Autodesk Fusion 360 part; units mm, degrees
note: some values were not read from the file. Set by a fixed rule: which sketch regions a step uses.
(part 4 of 5)
  spline S974 degree 3 poles (-10.77395, -44.821587) (-10.585081, -45.023839) (-10.376922, -45.203062) (-10.149782, -45.360193) knots 0 0 0 0 1 1 1 1
  spline S975 degree 3 poles (-10.149782, -45.359877) (-9.922331, -45.517324) (-9.680879, -45.648629) (-9.425424, -45.753798) knots 0 0 0 0 1 1 1 1
  spline S976 degree 3 poles (-9.425424, -45.753482) (-9.169969, -45.858967) (-8.906426, -45.936132) (-8.63448, -45.984667) knots 0 0 0 0 1 1 1 1
  spline S977 degree 3 poles (-8.63448, -45.984667) (-8.383382, -46.030411) (-8.130417, -46.050946) (-7.875585, -46.046586) knots 0 0 0 0 1 1 1 1
  spline S978 degree 3 poles (-7.875585, -46.046586) (-7.62013, -46.04099) (-7.368098, -46.010808) (-7.119178, -45.955112) knots 0 0 0 0 1 1 1 1
  spline S979 degree 3 poles (-7.119178, -45.955112) (-6.869947, -45.899727) (-6.628805, -45.820073) (-6.395754, -45.716149) knots 0 0 0 0 1 1 1 1
  spline S980 degree 3 poles (-6.395754, -45.716149) (-6.162391, -45.612225) (-5.942097, -45.486209) (-5.733937, -45.338101) knots 0 0 0 0 1 1 1 1
  spline S981 degree 3 poles (-5.733937, -45.338101) (-5.522666, -45.186571) (-5.328197, -45.016061) (-5.150219, -44.826259) knots 0 0 0 0 1 1 1 1
  spline S982 degree 3 poles (-5.150219, -44.826259) (-4.972552, -44.636457) (-4.814799, -44.431098) (-4.67727, -44.210181) knots 0 0 0 0 1 1 1 1
  spline S983 degree 3 poles (-4.67727, -44.210181) (-4.540053, -43.989265) (-4.425238, -43.757147) (-4.333449, -43.513827) knots 0 0 0 0 1 1 1 1
  spline S984 degree 3 poles (-4.333449, -43.513827) (-4.24166, -43.270196) (-4.174451, -43.020343) (-4.131824, -42.763644) knots 0 0 0 0 1 1 1 1
  spline S985 degree 3 poles (-4.131824, -42.763644) (-4.031011, -42.270782) (-3.876369, -41.795655) (-3.66821, -41.337953) knots 0 0 0 0 1 1 1 1
  spline S986 degree 3 poles (-3.66821, -41.337953) (-3.46005, -40.87994) (-3.203351, -40.451486) (-2.898113, -40.051658) knots 0 0 0 0 1 1 1 1
  line L17 (-2.898113, -40.051658) -> (-2.628968, -39.723701)
  spline S987 degree 3 poles (-2.628968, -39.723701) (-2.587897, -39.676095) (-2.537801, -39.641557) (-2.478683, -39.62071) knots 0 0 0 0 1 1 1 1
  spline S988 degree 3 poles (-2.478683, -39.62071) (-2.419564, -39.599863) (-2.35889, -39.595195) (-2.297282, -39.607019) knots 0 0 0 0 1 1 1 1
  spline S989 degree 3 poles (-11.970634, -36.872008) (-11.933296, -36.878851) (-11.898136, -36.890988) (-11.865154, -36.908724) knots 0 0 0 0 1 1 1 1
  spline S990 degree 3 poles (-11.865154, -36.908724) (-11.831861, -36.926771) (-11.802301, -36.949485) (-11.776476, -36.976866) knots 0 0 0 0 1 1 1 1
  spline S991 degree 3 poles (-11.776476, -36.976866) (-11.75065, -37.004247) (-11.729492, -37.035051) (-11.713623, -37.069277) knots 0 0 0 0 1 1 1 1
  spline S992 degree 3 poles (-11.713623, -37.069277) (-11.697444, -37.103504) (-11.687176, -37.139286) (-11.68282, -37.176624) knots 0 0 0 0 1 1 1 1
  line L18 (-11.68282, -37.176624) -> (-11.521333, -38.552842)
  spline S993 degree 3 poles (-11.521333, -38.552842) (-11.49893, -39.47478) (-11.568316, -40.389873) (-11.729181, -41.298121) knots 0 0 0 0 1 1 1 1
  line L19 (-11.729181, -41.298121) -> (-11.758429, -41.485433)
  spline S994 degree 3 poles (-11.758429, -41.485433) (-11.837772, -41.923533) (-11.842128, -42.362255) (-11.770564, -42.80191) knots 0 0 0 0 1 1 1 1
  spline S995 degree 3 poles (-11.770564, -42.80191) (-11.76745, -42.824313) (-11.766518, -42.847027) (-11.768386, -42.869119) knots 0 0 0 0 1 1 1 1
  spline S996 degree 3 poles (-11.768386, -42.869119) (-11.769002, -42.892455) (-11.772427, -42.914858) (-11.778028, -42.93695) knots 0 0 0 0 1 1 1 1
  spline S997 degree 3 poles (-11.778654, -42.936327) (-11.783627, -42.959041) (-11.791096, -42.980511) (-11.801053, -43.001047) knots 0 0 0 0 1 1 1 1
  spline S998 degree 3 poles (-11.801368, -43.000113) (-11.810699, -43.021582) (-11.822211, -43.041185) (-11.835591, -43.059543) knots 0 0 0 0 1 1 1 1
  spline S999 degree 3 poles (-11.835591, -43.059543) (-11.849281, -43.077901) (-11.864216, -43.094703) (-11.881645, -43.109327) knots 0 0 0 0 1 1 1 1
  spline S1000 degree 3 poles (-11.881645, -43.109327) (-11.897821, -43.125507) (-11.915867, -43.139197) (-11.93547, -43.151021) knots 0 0 0 0 1 1 1 1
  spline S1001 degree 3 poles (-11.93547, -43.151021) (-11.954761, -43.162845) (-11.975297, -43.172801) (-11.997081, -43.179958) knots 0 0 0 0 1 1 1 1
  spline S1002 degree 3 poles (-11.997081, -43.179958) (-12.017925, -43.18867) (-12.039705, -43.194582) (-12.062108, -43.198005) knots 0 0 0 0 1 1 1 1
  spline S1003 degree 3 poles (-12.062734, -43.197382) (-12.084511, -43.201741) (-12.107225, -43.203294) (-12.129939, -43.202672) knots 0 0 0 0 1 1 1 1
  spline S1004 degree 3 poles (-12.129939, -43.202672) (-12.152653, -43.201741) (-12.175056, -43.198936) (-12.197147, -43.19396) knots 0 0 0 0 1 1 1 1
  spline S1005 degree 3 poles (-12.197147, -43.19396) (-12.21955, -43.18867) (-12.241019, -43.181514) (-12.261555, -43.17249) knots 0 0 0 0 1 1 1 1
  spline S1006 degree 3 poles (-12.261555, -43.17249) (-12.282402, -43.163156) (-12.302005, -43.151954) (-12.320674, -43.138886) knots 0 0 0 0 1 1 1 1
  spline S1007 degree 3 poles (-12.320674, -43.138886) (-12.339343, -43.125818) (-12.356456, -43.111194) (-12.372325, -43.094703) knots 0 0 0 0 1 1 1 1
  spline S1008 degree 3 poles (-12.372325, -43.094703) (-12.387882, -43.078212) (-12.402195, -43.060476) (-12.414956, -43.040563) knots 0 0 0 0 1 1 1 1
  spline S1009 degree 3 poles (-12.414956, -43.040563) (-12.426776, -43.022205) (-12.437044, -43.00198) (-12.445445, -42.980822) knots 0 0 0 0 1 1 1 1
  spline S1010 degree 3 poles (-12.445445, -42.980822) (-12.453846, -42.959664) (-12.460069, -42.937883) (-12.464114, -42.91548) knots 0 0 0 0 1 1 1 1
  spline S1011 degree 3 poles (-12.464114, -42.91548) (-12.548747, -42.399593) (-12.545013, -41.884639) (-12.452605, -41.369997) knots 0 0 0 0 1 1 1 1
  line L20 (-12.452605, -41.369997) -> (-12.424602, -41.188285)
  spline S1012 degree 3 poles (-12.424602, -41.188285) (-12.271827, -40.3348) (-12.204307, -39.47478) (-12.221732, -38.607916) knots 0 0 0 0 1 1 1 1
  line L21 (-12.221732, -38.607916) -> (-12.383219, -37.259701)
  spline S1013 degree 3 poles (-12.383219, -37.259701) (-12.386333, -37.23232) (-12.386644, -37.204939) (-12.383537, -37.177869) knots 0 0 0 0 1 1 1 1
  spline S1014 degree 3 poles (-12.383537, -37.177869) (-12.380423, -37.150488) (-12.374203, -37.123729) (-12.364557, -37.097903) knots 0 0 0 0 1 1 1 1
  spline S1015 degree 3 poles (-12.364557, -37.097903) (-12.355223, -37.072078) (-12.343088, -37.047497) (-12.327841, -37.024472) knots 0 0 0 0 1 1 1 1
  spline S1016 degree 3 poles (-12.327841, -37.024472) (-12.312906, -37.001447) (-12.295482, -36.9806) (-12.275257, -36.961619) knots 0 0 0 0 1 1 1 1
  spline S1017 degree 3 poles (-12.275257, -36.961619) (-12.255343, -36.942639) (-12.233252, -36.926459) (-12.209604, -36.912769) knots 0 0 0 0 1 1 1 1
  spline S1018 degree 3 poles (-12.209604, -36.912769) (-12.185646, -36.898767) (-12.160754, -36.888188) (-12.134306, -36.880409) knots 0 0 0 0 1 1 1 1
  spline S1019 degree 3 poles (-12.134306, -36.880409) (-12.107858, -36.872319) (-12.081099, -36.867652) (-12.053718, -36.866096) knots 0 0 0 0 1 1 1 1
  spline S1020 degree 3 poles (-12.053718, -36.866096) (-12.026026, -36.864543) (-11.998956, -36.866415) (-11.971885, -36.871075) knots 0 0 0 0 1 1 1 1
  line L22 (-11.971885, -36.871075) -> (-11.970634, -36.872008)
  spline S1021 degree 3 poles (-10.675626, -35.450051) (-10.638599, -35.456583) (-10.603439, -35.46872) (-10.570457, -35.486456) knots 0 0 0 0 1 1 1 1
  spline S1022 degree 3 poles (-10.570457, -35.486456) (-10.537475, -35.504191) (-10.507916, -35.526905) (-10.482091, -35.553976) knots 0 0 0 0 1 1 1 1
  spline S1023 degree 3 poles (-10.482091, -35.553976) (-10.456265, -35.581357) (-10.435418, -35.611849) (-10.419238, -35.646076) knots 0 0 0 0 1 1 1 1
  spline S1024 degree 3 poles (-10.419238, -35.646076) (-10.403058, -35.679991) (-10.39279, -35.715463) (-10.388123, -35.752801) knots 0 0 0 0 1 1 1 1
  line L23 (-10.388123, -35.752801) -> (-10.25215, -36.838404)
  spline S1025 degree 3 poles (-10.25215, -36.838404) (-10.073861, -38.475054) (-10.114622, -40.106104) (-10.375052, -41.732173) knots 0 0 0 0 1 1 1 1
  spline S1026 degree 3 poles (-10.375052, -41.732173) (-10.388434, -41.811208) (-10.39808, -41.891173) (-10.403682, -41.971761) knots 0 0 0 0 1 1 1 1
  spline S1027 degree 3 poles (-10.403989, -41.972381) (-10.409281, -42.052349) (-10.411146, -42.132937) (-10.408971, -42.213525) knots 0 0 0 0 1 1 1 1
  spline S1028 degree 3 poles (-10.408968, -42.214145) (-10.406797, -42.294113) (-10.40057, -42.374701) (-10.390614, -42.454667) knots 0 0 0 0 1 1 1 1
  spline S1029 degree 3 poles (-10.39061, -42.455286) (-10.380346, -42.534943) (-10.366344, -42.614287) (-10.348608, -42.693008) knots 0 0 0 0 1 1 1 1
  spline S1030 degree 3 poles (-10.348605, -42.693628) (-10.330562, -42.771729) (-10.309092, -42.849205) (-10.283578, -42.925748) knots 0 0 0 0 1 1 1 1
  spline S1031 degree 3 poles (-10.283574, -42.926368) (-10.258064, -43.002291) (-10.228815, -43.077589) (-10.195834, -43.151332) knots 0 0 0 0 1 1 1 1
  spline S1032 degree 3 poles (-10.19583, -43.151952) (-10.162852, -43.224764) (-10.126447, -43.296639) (-10.08662, -43.366959) knots 0 0 0 0 1 1 1 1
  spline S1033 degree 3 poles (-10.086616, -43.367579) (-10.046793, -43.436968) (-10.003543, -43.504799) (-9.95687, -43.570763) knots 0 0 0 0 1 1 1 1
  spline S1034 degree 3 poles (-9.956866, -43.571383) (-9.910198, -43.636727) (-9.860413, -43.69989) (-9.807518, -43.760876) knots 0 0 0 0 1 1 1 1
  spline S1035 degree 3 poles (-9.807825, -43.761495) (-9.754622, -43.821861) (-9.698926, -43.880046) (-9.64043, -43.935431) knots 0 0 0 0 1 1 1 1
  spline S1036 degree 3 poles (-9.640738, -43.936362) (-9.581934, -43.991127) (-9.520949, -44.0434) (-9.457163, -44.092873) knots 0 0 0 0 1 1 1 1
  spline S1037 degree 3 poles (-9.457159, -44.093493) (-9.393377, -44.142346) (-9.327413, -44.188396) (-9.259271, -44.231335) knots 0 0 0 0 1 1 1 1
  spline S1038 degree 3 poles (-9.259267, -44.232266) (-9.190818, -44.274273) (-9.120809, -44.31379) (-9.048622, -44.349883) knots 0 0 0 0 1 1 1 1
  spline S1039 degree 3 poles (-9.048619, -44.350503) (-8.976436, -44.385976) (-8.902693, -44.418336) (-8.827395, -44.446962) knots 0 0 0 0 1 1 1 1
  spline S1040 degree 3 poles (-8.827702, -44.447893) (-8.752096, -44.475899) (-8.675553, -44.500791) (-8.597766, -44.52226) knots 0 0 0 0 1 1 1 1
  spline S1041 degree 3 poles (-8.598073, -44.52288) (-8.519978, -44.543418) (-8.441568, -44.560843) (-8.361914, -44.574222) knots 0 0 0 0 1 1 1 1
  spline S1042 degree 3 poles (-8.362221, -44.574842) (-8.28257, -44.587602) (-8.202605, -44.597247) (-8.122017, -44.602848) knots 0 0 0 0 1 1 1 1
  spline S1043 degree 3 poles (-8.122324, -44.603779) (-8.04174, -44.608449) (-7.961152, -44.610311) (-7.880564, -44.608138) knots 0 0 0 0 1 1 1 1
  spline S1044 degree 3 poles (-7.880872, -44.608758) (-7.799978, -44.605653) (-7.7197, -44.599426) (-7.639734, -44.589158) knots 0 0 0 0 1 1 1 1
  spline S1045 degree 3 poles (-7.640041, -44.590089) (-7.559768, -44.579201) (-7.480425, -44.564888) (-7.402014, -44.547152) knots 0 0 0 0 1 1 1 1
  spline S1046 degree 3 poles (-7.402011, -44.547772) (-7.323293, -44.529106) (-7.245818, -44.507325) (-7.169275, -44.4815) knots 0 0 0 0 1 1 1 1
  spline S1047 degree 3 poles (-7.169582, -44.482431) (-7.093043, -44.455985) (-7.017744, -44.426737) (-6.944313, -44.393755) knots 0 0 0 0 1 1 1 1
  spline S1048 degree 3 poles (-6.94431, -44.394375) (-6.87057, -44.360773) (-6.799006, -44.324058) (-6.728996, -44.28423) knots 0 0 0 0 1 1 1 1
  spline S1049 degree 3 poles (-6.728993, -44.28485) (-6.658988, -44.244092) (-6.591157, -44.200531) (-6.525194, -44.153858) knots 0 0 0 0 1 1 1 1
  spline S1050 degree 3 poles (-6.525502, -44.154478) (-6.459541, -44.107186) (-6.396066, -44.057402) (-6.335392, -44.004195) knots 0 0 0 0 1 1 1 1
  spline S1051 degree 3 poles (-6.335389, -44.005126) (-6.274406, -43.951299) (-6.216221, -43.895604) (-6.160837, -43.836796) knots 0 0 0 0 1 1 1 1
  spline S1052 degree 3 poles (-6.161145, -43.837416) (-6.105452, -43.777989) (-6.053179, -43.717003) (-6.003706, -43.652906) knots 0 0 0 0 1 1 1 1
  spline S1053 degree 3 poles (-6.004014, -43.653837) (-5.954545, -43.589121) (-5.908494, -43.523157) (-5.865555, -43.454704) knots 0 0 0 0 1 1 1 1
  spline S1054 degree 3 poles (-5.865552, -43.455323) (-5.822616, -43.386251) (-5.7831, -43.315931) (-5.747007, -43.243744) knots 0 0 0 0 1 1 1 1
  spline S1055 degree 3 poles (-5.747315, -43.244364) (-5.711224, -43.171557) (-5.678865, -43.097814) (-5.649928, -43.022205) knots 0 0 0 0 1 1 1 1
  spline S1056 degree 3 poles (-5.650237, -43.022825) (-5.621301, -42.946906) (-5.596409, -42.870052) (-5.575252, -42.792265) knots 0 0 0 0 1 1 1 1
  spline S1057 degree 3 poles (-5.575249, -42.792885) (-5.553782, -42.714477) (-5.536668, -42.635756) (-5.522978, -42.556102) knots 0 0 0 0 1 1 1 1
  spline S1058 degree 3 poles (-5.523287, -42.556721) (-5.431811, -42.127959) (-5.309218, -41.709151) (-5.15551, -41.299366) knots 0 0 0 0 1 1 1 1
  spline S1059 degree 3 poles (-5.155819, -41.299985) (-5.001802, -40.889892) (-4.818845, -40.493797) (-4.606019, -40.111083) knots 0 0 0 0 1 1 1 1
  spline S1060 degree 3 poles (-4.606327, -40.111391) (-4.393503, -39.728679) (-4.153917, -39.364011) (-3.887261, -39.017389) knots 0 0 0 0 1 1 1 1
  spline S1061 degree 3 poles (-3.887259, -39.017698) (-3.620294, -38.670768) (-3.329369, -38.345616) (-3.014171, -38.042242) knots 0 0 0 0 1 1 1 1
  spline S1062 degree 3 poles (-3.014171, -38.042242) (-2.997994, -38.025753) (-2.980258, -38.011129) (-2.961276, -37.99837) knots 0 0 0 0 1 1 1 1
  spline S1063 degree 3 poles (-2.961276, -37.99837) (-2.941987, -37.985304) (-2.921762, -37.974414) (-2.90029, -37.965699) knots 0 0 0 0 1 1 1 1
  spline S1064 degree 3 poles (-2.90029, -37.965699) (-2.879134, -37.956678) (-2.857043, -37.949833) (-2.834638, -37.945474) knots 0 0 0 0 1 1 1 1
  spline S1065 degree 3 poles (-2.834638, -37.945474) (-2.811926, -37.940809) (-2.788901, -37.938634) (-2.765873, -37.93832) knots 0 0 0 0 1 1 1 1
  spline S1066 degree 3 poles (-2.765873, -37.93832) (-2.742851, -37.938323) (-2.719826, -37.940498) (-2.69742, -37.945163) knots 0 0 0 0 1 1 1 1
  spline S1067 degree 3 poles (-2.69742, -37.945163) (-2.674709, -37.949522) (-2.652617, -37.956056) (-2.631145, -37.964766) knots 0 0 0 0 1 1 1 1
  spline S1068 degree 3 poles (-2.631145, -37.964766) (-2.609989, -37.973791) (-2.589765, -37.98437) (-2.570471, -37.997125) knots 0 0 0 0 1 1 1 1
  spline S1069 degree 3 poles (-2.570471, -37.997125) (-2.551182, -38.010196) (-2.533447, -38.024509) (-2.516953, -38.040997) knots 0 0 0 0 1 1 1 1
  spline S1070 degree 3 poles (-2.516953, -38.040997) (-2.500776, -38.05718) (-2.486152, -38.074915) (-2.473081, -38.094204) knots 0 0 0 0 1 1 1 1
  spline S1071 degree 3 poles (-2.473081, -38.094204) (-2.460326, -38.113187) (-2.449436, -38.133723) (-2.440721, -38.154878) knots 0 0 0 0 1 1 1 1
  spline S1072 degree 3 poles (-2.440721, -38.154878) (-2.4317, -38.17635) (-2.424855, -38.198131) (-2.420497, -38.220842) knots 0 0 0 0 1 1 1 1
  spline S1073 degree 3 poles (-2.420497, -38.220842) (-2.415832, -38.243559) (-2.413654, -38.266584) (-2.413651, -38.289606) knots 0 0 0 0 1 1 1 1
  spline S1074 degree 3 poles (-2.413651, -38.289606) (-2.413343, -38.312634) (-2.415521, -38.335659) (-2.420185, -38.358371) knots 0 0 0 0 1 1 1 1
  spline S1075 degree 3 poles (-2.420185, -38.358371) (-2.424544, -38.381087) (-2.431078, -38.402868) (-2.440099, -38.424334) knots 0 0 0 0 1 1 1 1
  spline S1076 degree 3 poles (-2.440099, -38.424334) (-2.448814, -38.445806) (-2.459393, -38.466031) (-2.472459, -38.48532) knots 0 0 0 0 1 1 1 1
  spline S1077 degree 3 poles (-2.472459, -38.48532) (-2.485218, -38.504614) (-2.499531, -38.522349) (-2.51602, -38.538838) knots 0 0 0 0 1 1 1 1
  spline S1078 degree 3 poles (-2.51602, -38.538838) (-2.804458, -38.817009) (-3.070803, -39.114779) (-3.315676, -39.43215) knots 0 0 0 0 1 1 1 1
  spline S1079 degree 3 poles (-3.315676, -39.43215) (-3.560554, -39.749526) (-3.780848, -40.083079) (-3.976559, -40.43281) knots 0 0 0 0 1 1 1 1
  spline S1080 degree 3 poles (-3.976559, -40.43281) (-4.172586, -40.782545) (-4.341852, -41.144724) (-4.484668, -41.519346) knots 0 0 0 0 1 1 1 1
  spline S1081 degree 3 poles (-4.484668, -41.519346) (-4.627488, -41.893974) (-4.742302, -42.277) (-4.829111, -42.668424) knots 0 0 0 0 1 1 1 1
  spline S1082 degree 3 poles (-4.829111, -42.668424) (-4.846227, -42.770795) (-4.868629, -42.871919) (-4.895697, -42.972107) knots 0 0 0 0 1 1 1 1
  spline S1083 degree 3 poles (-4.895697, -42.972107) (-4.92277, -43.0723) (-4.954818, -43.170935) (-4.991843, -43.2677) knots 0 0 0 0 1 1 1 1
  spline S1084 degree 3 poles (-4.991843, -43.2677) (-5.028561, -43.364781) (-5.069944, -43.459682) (-5.116303, -43.552714) knots 0 0 0 0 1 1 1 1
  spline S1085 degree 3 poles (-5.116303, -43.552714) (-5.162355, -43.64575) (-5.213073, -43.735983) (-5.268144, -43.824037) knots 0 0 0 0 1 1 1 1
  spline S1086 degree 3 poles (-5.268144, -43.824037) (-5.322909, -43.911783) (-5.382339, -43.997039) (-5.4455, -44.07918) knots 0 0 0 0 1 1 1 1
  spline S1087 degree 3 poles (-5.4455, -44.07918) (-5.508978, -44.161326) (-5.576186, -44.240047) (-5.647436, -44.315654) knots 0 0 0 0 1 1 1 1
  spline S1088 degree 3 poles (-5.647436, -44.315654) (-5.718381, -44.390955) (-5.793058, -44.462831) (-5.871153, -44.53097) knots 0 0 0 0 1 1 1 1
  spline S1089 degree 3 poles (-5.871153, -44.53097) (-5.949256, -44.599114) (-6.030777, -44.663522) (-6.115095, -44.723572) knots 0 0 0 0 1 1 1 1
  spline S1090 degree 3 poles (-6.115095, -44.723572) (-6.199421, -44.783627) (-6.286854, -44.839634) (-6.376772, -44.891282) knots 0 0 0 0 1 1 1 1
  spline S1091 degree 3 poles (-6.376772, -44.891282) (-6.466699, -44.942935) (-6.558799, -44.989919) (-6.653386, -45.032544) knots 0 0 0 0 1 1 1 1
  spline S1092 degree 3 poles (-6.653386, -45.032544) (-6.747978, -45.074863) (-6.844124, -45.112824) (-6.942444, -45.145803) knots 0 0 0 0 1 1 1 1
  spline S1093 degree 3 poles (-6.942444, -45.145803) (-7.040771, -45.178787) (-7.140339, -45.207102) (-7.24146, -45.230125) knots 0 0 0 0 1 1 1 1
  spline S1094 degree 3 poles (-7.24146, -45.230125) (-7.342275, -45.253463) (-7.444333, -45.271821) (-7.547009, -45.284887) knots 0 0 0 0 1 1 1 1
  spline S1095 degree 3 poles (-7.547009, -45.284887) (-7.649692, -45.298269) (-7.752994, -45.306359) (-7.856603, -45.309468) knots 0 0 0 0 1 1 1 1
  spline S1096 degree 3 poles (-7.856603, -45.309468) (-7.96022, -45.312584) (-8.063522, -45.310402) (-8.16682, -45.303247) knots 0 0 0 0 1 1 1 1
  spline S1097 degree 3 poles (-8.16682, -45.303247) (-8.270438, -45.296089) (-8.373116, -45.283959) (-8.47517, -45.266843) knots 0 0 0 0 1 1 1 1
  spline S1098 degree 3 poles (-8.47517, -45.266843) (-8.577542, -45.249732) (-8.678666, -45.227329) (-8.778542, -45.200257) knots 0 0 0 0 1 1 1 1
  spline S1099 degree 3 poles (-8.778542, -45.200257) (-8.878424, -45.173189) (-8.977059, -45.141141) (-9.073823, -45.104422) knots 0 0 0 0 1 1 1 1
  spline S1100 degree 3 poles (-9.073823, -45.104422) (-9.170595, -45.067398) (-9.265495, -45.026015) (-9.358215, -44.979651) knots 0 0 0 0 1 1 1 1
  spline S1101 degree 3 poles (-9.358215, -44.979651) (-9.450941, -44.933603) (-9.541175, -44.882886) (-9.628915, -44.82781) knots 0 0 0 0 1 1 1 1
  spline S1102 degree 3 poles (-9.628915, -44.82781) (-9.716974, -44.772739) (-9.801607, -44.71362) (-9.883747, -44.650143) knots 0 0 0 0 1 1 1 1
  spline S1103 degree 3 poles (-9.883747, -44.650143) (-9.965584, -44.586671) (-10.044305, -44.519462) (-10.11991, -44.448206) knots 0 0 0 0 1 1 1 1
  spline S1104 degree 3 poles (-10.11991, -44.448206) (-10.195212, -44.377267) (-10.266777, -44.302591) (-10.334914, -44.224178) knots 0 0 0 0 1 1 1 1
  spline S1105 degree 3 poles (-10.334914, -44.224178) (-10.40306, -44.146082) (-10.466845, -44.064561) (-10.526894, -43.980236) knots 0 0 0 0 1 1 1 1
  spline S1106 degree 3 poles (-10.526894, -43.980236) (-10.586949, -43.895606) (-10.642956, -43.808484) (-10.694293, -43.718248) knots 0 0 0 0 1 1 1 1
  spline S1107 degree 3 poles (-10.694293, -43.718248) (-10.745947, -43.628328) (-10.792931, -43.535916) (-10.835244, -43.441324) knots 0 0 0 0 1 1 1 1
  spline S1108 degree 3 poles (-10.835244, -43.441324) (-10.877564, -43.346737) (-10.915213, -43.25028) (-10.948191, -43.151954) knots 0 0 0 0 1 1 1 1
  spline S1109 degree 3 poles (-10.948191, -43.151954) (-10.981177, -43.053633) (-11.009492, -42.953754) (-11.032513, -42.852628) knots 0 0 0 0 1 1 1 1
  spline S1110 degree 3 poles (-11.032513, -42.852628) (-11.055542, -42.751506) (-11.0739, -42.649449) (-11.086964, -42.546456) knots 0 0 0 0 1 1 1 1
  spline S1111 degree 3 poles (-11.086964, -42.546456) (-11.100036, -42.443779) (-11.108126, -42.340477) (-11.111234, -42.23655) knots 0 0 0 0 1 1 1 1
  spline S1112 degree 3 poles (-11.111234, -42.23655) (-11.114352, -42.13294) (-11.11217, -42.029327) (-11.105013, -41.925711) knots 0 0 0 0 1 1 1 1
  spline S1113 degree 3 poles (-11.105013, -41.925711) (-11.097864, -41.822412) (-11.085726, -41.719421) (-11.068609, -41.61705) knots 0 0 0 0 1 1 1 1
  spline S1114 degree 3 poles (-11.068609, -41.61705) (-10.819692, -40.059434) (-10.780798, -38.496837) (-10.95162, -36.928951) knots 0 0 0 0 1 1 1 1
  line L24 (-10.95162, -36.928951) -> (-11.0879, -35.84054)
  spline S1115 degree 3 poles (-11.0879, -35.84054) (-11.090704, -35.81752) (-11.091325, -35.794495) (-11.089765, -35.771465) knots 0 0 0 0 1 1 1 1
  spline S1116 degree 3 poles (-11.089765, -35.771465) (-11.088211, -35.748444) (-11.084165, -35.72573) (-11.078252, -35.703323) knots 0 0 0 0 1 1 1 1
  spline S1117 degree 3 poles (-11.078252, -35.703323) (-11.072032, -35.681236) (-11.063939, -35.659767) (-11.05336, -35.638915) knots 0 0 0 0 1 1 1 1
  spline S1118 degree 3 poles (-11.05336, -35.638915) (-11.043092, -35.618384) (-11.030957, -35.598781) (-11.016644, -35.580418) knots 0 0 0 0 1 1 1 1
  spline S1119 degree 3 poles (-11.016644, -35.580418) (-11.002643, -35.562377) (-10.986774, -35.545574) (-10.969349, -35.530323) knots 0 0 0 0 1 1 1 1
  spline S1120 degree 3 poles (-10.969349, -35.530323) (-10.951925, -35.515393) (-10.932945, -35.502013) (-10.913031, -35.490496) knots 0 0 0 0 1 1 1 1
  spline S1121 degree 3 poles (-10.913031, -35.490496) (-10.893118, -35.479299) (-10.871959, -35.469654) (-10.850179, -35.462492) knots 0 0 0 0 1 1 1 1
  spline S1122 degree 3 poles (-10.850179, -35.462492) (-10.828087, -35.455035) (-10.805684, -35.450051) (-10.78297, -35.447246) knots 0 0 0 0 1 1 1 1
  spline S1123 degree 3 poles (-10.78297, -35.447246) (-10.746877, -35.442584) (-10.711095, -35.443515) (-10.675626, -35.450051) knots 0 0 0 0 1 1 1 1
  spline S1124 degree 3 poles (-5.153642, -34.44877) (-5.0883, -34.460593) (-5.030738, -34.488597) (-4.980953, -34.533091) knots 0 0 0 0 1 1 1 1
  spline S1125 degree 3 poles (-4.980953, -34.533091) (-4.931481, -34.577586) (-4.897254, -34.631726) (-4.878585, -34.695512) knots 0 0 0 0 1 1 1 1
  spline S1126 degree 3 poles (-4.878585, -34.695512) (-4.859605, -34.759609) (-4.858983, -34.823706) (-4.876407, -34.887803) knots 0 0 0 0 1 1 1 1
  spline S1127 degree 3 poles (-4.876407, -34.887803) (-4.894143, -34.952211) (-4.927124, -35.007284) (-4.975975, -35.052712) knots 0 0 0 0 1 1 1 1
  spline S1128 degree 3 poles (-4.975975, -35.052712) (-5.485639, -35.502947) (-5.956098, -35.991142) (-6.387042, -36.517297) knots 0 0 0 0 1 1 1 1
  spline S1129 degree 3 poles (-6.387042, -36.517297) (-6.817984, -37.043452) (-7.204122, -37.601033) (-7.546388, -38.189421) knots 0 0 0 0 1 1 1 1
  spline S1130 degree 3 poles (-7.546388, -38.189421) (-7.886474, -38.778115) (-8.178334, -39.390459) (-8.420719, -40.026139) knots 0 0 0 0 1 1 1 1
  spline S1131 degree 3 poles (-8.421342, -40.026141) (-8.663416, -40.661819) (-8.853218, -41.313056) (-8.990747, -41.979231) knots 0 0 0 0 1 1 1 1
  spline S1132 degree 3 poles (-8.990747, -41.979231) (-9.003192, -42.047682) (-9.009104, -42.116446) (-9.00786, -42.185835) knots 0 0 0 0 1 1 1 1
  spline S1133 degree 3 poles (-9.00786, -42.185835) (-9.006927, -42.254908) (-8.999147, -42.323672) (-8.984524, -42.391506) knots 0 0 0 0 1 1 1 1
  spline S1134 degree 3 poles (-8.984524, -42.391506) (-8.969899, -42.459334) (-8.949052, -42.524987) (-8.921672, -42.588464) knots 0 0 0 0 1 1 1 1
  spline S1135 degree 3 poles (-8.921672, -42.588464) (-8.893978, -42.652247) (-8.860685, -42.71261) (-8.82117, -42.769553) knots 0 0 0 0 1 1 1 1
  spline S1136 degree 3 poles (-8.82117, -42.769553) (-8.781964, -42.826802) (-8.73747, -42.879387) (-8.687687, -42.927617) knots 0 0 0 0 1 1 1 1
  spline S1137 degree 3 poles (-8.687687, -42.927617) (-8.637902, -42.975843) (-8.584073, -43.018782) (-8.525889, -43.056434) knots 0 0 0 0 1 1 1 1
  spline S1138 degree 3 poles (-8.525889, -43.056434) (-8.467702, -43.09408) (-8.406406, -43.125507) (-8.341999, -43.151023) knots 0 0 0 0 1 1 1 1
  spline S1139 degree 3 poles (-8.341999, -43.151023) (-8.27759, -43.176535) (-8.211315, -43.195515) (-8.143174, -43.207964) knots 0 0 0 0 1 1 1 1
  spline S1140 degree 3 poles (-8.143174, -43.207964) (-8.075031, -43.220407) (-8.006267, -43.226319) (-7.937192, -43.225077) knots 0 0 0 0 1 1 1 1
  spline S1141 degree 3 poles (-7.937192, -43.225077) (-7.867805, -43.223833) (-7.799352, -43.216051) (-7.731522, -43.20143) knots 0 0 0 0 1 1 1 1
  spline S1142 degree 3 poles (-7.731522, -43.20143) (-7.664001, -43.186803) (-7.598348, -43.165645) (-7.534564, -43.138266) knots 0 0 0 0 1 1 1 1
  spline S1143 degree 3 poles (-7.534564, -43.138266) (-7.471088, -43.110571) (-7.410725, -43.076967) (-7.353786, -43.037765) knots 0 0 0 0 1 1 1 1
  spline S1144 degree 3 poles (-7.353786, -43.037765) (-7.296844, -42.998246) (-7.244259, -42.953441) (-7.196034, -42.903659) knots 0 0 0 0 1 1 1 1
  spline S1145 degree 3 poles (-7.196034, -42.903659) (-7.147803, -42.853872) (-7.105175, -42.799732) (-7.067528, -42.74155) knots 0 0 0 0 1 1 1 1
  spline S1146 degree 3 poles (-7.067528, -42.74155) (-7.029878, -42.683362) (-6.998451, -42.621754) (-6.972938, -42.557349) knots 0 0 0 0 1 1 1 1
  spline S1147 degree 3 poles (-6.972938, -42.557349) (-6.947422, -42.492938) (-6.928442, -42.426352) (-6.915998, -42.358212) knots 0 0 0 0 1 1 1 1
  spline S1148 degree 3 poles (-6.915998, -42.358212) (-6.801181, -41.805296) (-6.642495, -41.265139) (-6.439316, -40.738053) knots 0 0 0 0 1 1 1 1
  spline S1149 degree 3 poles (-6.439316, -40.738053) (-6.237066, -40.210962) (-5.993124, -39.703787) (-5.70811, -39.216526) knots 0 0 0 0 1 1 1 1
  spline S1150 degree 3 poles (-5.707179, -39.216528) (-5.422786, -38.729264) (-5.100123, -38.268139) (-4.740122, -37.833463) knots 0 0 0 0 1 1 1 1
  spline S1151 degree 3 poles (-4.740122, -37.833463) (-4.37981, -37.398474) (-3.986827, -36.995846) (-3.561173, -36.625266) knots 0 0 0 0 1 1 1 1
  spline S1152 degree 3 poles (-3.561173, -36.625266) (-3.54406, -36.61002) (-3.525702, -36.59664) (-3.5061, -36.585128) knots 0 0 0 0 1 1 1 1
  spline S1153 degree 3 poles (-3.5061, -36.585128) (-3.486186, -36.573615) (-3.46565, -36.564281) (-3.44387, -36.556813) knots 0 0 0 0 1 1 1 1
  spline S1154 degree 3 poles (-3.44387, -36.556813) (-3.4224, -36.549032) (-3.400309, -36.543745) (-3.377595, -36.540633) knots 0 0 0 0 1 1 1 1
  spline S1155 degree 3 poles (-3.377595, -36.540633) (-3.355192, -36.537519) (-3.332478, -36.536586) (-3.309453, -36.537838) knots 0 0 0 0 1 1 1 1
  spline S1156 degree 3 poles (-3.309453, -36.537838) (-3.286739, -36.538769) (-3.264336, -36.542505) (-3.242244, -36.548106) knots 0 0 0 0 1 1 1 1
  spline S1157 degree 3 poles (-3.242244, -36.548106) (-3.220153, -36.553706) (-3.198683, -36.561174) (-3.178147, -36.571131) knots 0 0 0 0 1 1 1 1
  spline S1158 degree 3 poles (-3.178147, -36.571131) (-3.1573, -36.580776) (-3.138009, -36.5926) (-3.119651, -36.606291) knots 0 0 0 0 1 1 1 1
  spline S1159 degree 3 poles (-3.119651, -36.606291) (-3.101293, -36.61967) (-3.08418, -36.634916) (-3.068934, -36.65203) knots 0 0 0 0 1 1 1 1
  spline S1160 degree 3 poles (-3.068934, -36.65203) (-3.053687, -36.668832) (-3.039997, -36.68719) (-3.028173, -36.706481) knots 0 0 0 0 1 1 1 1
  spline S1161 degree 3 poles (-3.028173, -36.706481) (-3.016349, -36.726084) (-3.006393, -36.746619) (-2.998614, -36.768089) knots 0 0 0 0 1 1 1 1
  spline S1162 degree 3 poles (-2.998614, -36.768089) (-2.990835, -36.789558) (-2.984923, -36.81165) (-2.981501, -36.834364) knots 0 0 0 0 1 1 1 1
  spline S1163 degree 3 poles (-2.981501, -36.834364) (-2.978078, -36.856767) (-2.976522, -36.879481) (-2.977456, -36.902506) knots 0 0 0 0 1 1 1 1
  spline S1164 degree 3 poles (-2.977456, -36.902506) (-2.978389, -36.92522) (-2.981501, -36.947934) (-2.98679, -36.970025) knots 0 0 0 0 1 1 1 1
  spline S1165 degree 3 poles (-2.98679, -36.970025) (-2.99208, -36.992428) (-2.999236, -37.013898) (-3.008882, -37.034745) knots 0 0 0 0 1 1 1 1
  spline S1166 degree 3 poles (-3.008882, -37.034745) (-3.018216, -37.055592) (-3.029729, -37.075194) (-3.042797, -37.093863) knots 0 0 0 0 1 1 1 1
  spline S1167 degree 3 poles (-3.042797, -37.093863) (-3.056177, -37.112532) (-3.071112, -37.129645) (-3.087603, -37.145203) knots 0 0 0 0 1 1 1 1
  spline S1168 degree 3 poles (-3.087603, -37.145203) (-3.482452, -37.49058) (-3.847121, -37.865205) (-4.181918, -38.269389) knots 0 0 0 0 1 1 1 1
  spline S1169 degree 3 poles (-4.181918, -38.269389) (-4.516405, -38.673262) (-4.816976, -39.101094) (-5.08239, -39.55319) knots 0 0 0 0 1 1 1 1
  spline S1170 degree 3 poles (-5.08239, -39.55319) (-5.349354, -40.005296) (-5.57805, -40.475756) (-5.768785, -40.964573) knots 0 0 0 0 1 1 1 1
  spline S1171 degree 3 poles (-5.768476, -40.964568) (-5.959831, -41.45339) (-6.11074, -41.954342) (-6.221511, -42.467113) knots 0 0 0 0 1 1 1 1
  spline S1172 degree 3 poles (-6.221511, -42.467113) (-6.231154, -42.524058) (-6.243911, -42.580065) (-6.25916, -42.635756) knots 0 0 0 0 1 1 1 1
  spline S1173 degree 3 poles (-6.25916, -42.635756) (-6.274715, -42.691146) (-6.292761, -42.745908) (-6.313611, -42.799732) knots 0 0 0 0 1 1 1 1
  spline S1174 degree 3 poles (-6.313611, -42.799732) (-6.334145, -42.853566) (-6.357792, -42.906151) (-6.38362, -42.957485) knots 0 0 0 0 1 1 1 1
  spline S1175 degree 3 poles (-6.38362, -42.957485) (-6.409443, -43.009141) (-6.437757, -43.058925) (-6.468564, -43.107771) knots 0 0 0 0 1 1 1 1
  spline S1176 degree 3 poles (-6.468564, -43.107771) (-6.499677, -43.156315) (-6.532658, -43.20361) (-6.568132, -43.249033) knots 0 0 0 0 1 1 1 1
  spline S1177 degree 3 poles (-6.568132, -43.249033) (-6.603601, -43.294466) (-6.64125, -43.338027) (-6.681079, -43.379716) knots 0 0 0 0 1 1 1 1
  spline S1178 degree 3 poles (-6.681079, -43.379716) (-6.720594, -43.421415) (-6.762287, -43.460931) (-6.805851, -43.498576) knots 0 0 0 0 1 1 1 1
  spline S1179 degree 3 poles (-6.805851, -43.498576) (-6.84972, -43.53623) (-6.894837, -43.571701) (-6.942134, -43.604989) knots 0 0 0 0 1 1 1 1
  spline S1180 degree 3 poles (-6.942134, -43.604989) (-6.989116, -43.637976) (-7.037654, -43.66878) (-7.087752, -43.697401) knots 0 0 0 0 1 1 1 1
  spline S1181 degree 3 poles (-7.087752, -43.697401) (-7.137845, -43.72572) (-7.189185, -43.751546) (-7.242083, -43.774877) knots 0 0 0 0 1 1 1 1
  spline S1182 degree 3 poles (-7.242083, -43.774877) (-7.294665, -43.798218) (-7.348182, -43.818754) (-7.402947, -43.837107) knots 0 0 0 0 1 1 1 1
  spline S1183 degree 3 poles (-7.402947, -43.837107) (-7.457707, -43.855159) (-7.513092, -43.870405) (-7.569102, -43.882846) knots 0 0 0 0 1 1 1 1
  spline S1184 degree 3 poles (-7.569102, -43.882846) (-7.625417, -43.895608) (-7.682045, -43.905254) (-7.739301, -43.912406) knots 0 0 0 0 1 1 1 1
  spline S1185 degree 3 poles (-7.739301, -43.912406) (-7.796238, -43.919565) (-7.8538, -43.923612) (-7.911056, -43.925163) knots 0 0 0 0 1 1 1 1
  spline S1186 degree 3 poles (-7.911056, -43.925163) (-7.968615, -43.92641) (-8.026178, -43.925168) (-8.083744, -43.920807) knots 0 0 0 0 1 1 1 1
  spline S1187 degree 3 poles (-8.083744, -43.920807) (-8.140992, -43.916456) (-8.198244, -43.909299) (-8.254877, -43.899649) knots 0 0 0 0 1 1 1 1
  spline S1188 degree 3 poles (-8.254877, -43.899649) (-8.311503, -43.889697) (-8.36751, -43.876939) (-8.423209, -43.861688) knots 0 0 0 0 1 1 1 1
  spline S1189 degree 3 poles (-8.423209, -43.861688) (-8.47859, -43.846136) (-8.533042, -43.828089) (-8.586874, -43.807548) knots 0 0 0 0 1 1 1 1
  spline S1190 degree 3 poles (-8.586874, -43.807548) (-8.640388, -43.786706) (-8.692973, -43.76337) (-8.744316, -43.737228) knots 0 0 0 0 1 1 1 1
  spline S1191 degree 3 poles (-8.744316, -43.737228) (-8.795964, -43.711407) (-8.845748, -43.683093) (-8.894291, -43.652284) knots 0 0 0 0 1 1 1 1
  spline S1192 degree 3 poles (-8.894291, -43.652284) (-8.943139, -43.621485) (-8.990121, -43.588192) (-9.035242, -43.552716) knots 0 0 0 0 1 1 1 1
  spline S1193 degree 3 poles (-9.035242, -43.552716) (-9.080667, -43.51725) (-9.124228, -43.479601) (-9.165925, -43.439768) knots 0 0 0 0 1 1 1 1
  spline S1194 degree 3 poles (-9.165925, -43.439768) (-9.207617, -43.399946) (-9.247133, -43.358252) (-9.284784, -43.314686) knots 0 0 0 0 1 1 1 1
  spline S1195 degree 3 poles (-9.284784, -43.314686) (-9.322431, -43.27113) (-9.357591, -43.225702) (-9.390575, -43.178402) knots 0 0 0 0 1 1 1 1
  spline S1196 degree 3 poles (-9.390575, -43.178402) (-9.423865, -43.131423) (-9.45467, -43.082573) (-9.482987, -43.032473) knots 0 0 0 0 1 1 1 1
  spline S1197 degree 3 poles (-9.482987, -43.032473) (-9.511299, -42.982382) (-9.537125, -42.931043) (-9.560152, -42.878142) knots 0 0 0 0 1 1 1 1
  spline S1198 degree 3 poles (-9.560152, -42.878142) (-9.583486, -42.825563) (-9.604333, -42.771734) (-9.622382, -42.716966) knots 0 0 0 0 1 1 1 1
  spline S1199 degree 3 poles (-9.622382, -42.716966) (-9.640115, -42.662209) (-9.655673, -42.606824) (-9.668121, -42.550501) knots 0 0 0 0 1 1 1 1
  spline S1200 degree 3 poles (-9.668121, -42.550501) (-9.680565, -42.494499) (-9.690522, -42.437558) (-9.69737, -42.380302) knots 0 0 0 0 1 1 1 1
  spline S1201 degree 3 poles (-9.69737, -42.380302) (-9.70452, -42.323366) (-9.708569, -42.265803) (-9.710127, -42.208236) knots 0 0 0 0 1 1 1 1
  spline S1202 degree 3 poles (-9.710127, -42.208236) (-9.711366, -42.150678) (-9.709806, -42.093115) (-9.705459, -42.035547) knots 0 0 0 0 1 1 1 1
  spline S1203 degree 3 poles (-9.705459, -42.035547) (-9.701411, -41.977989) (-9.694256, -41.921049) (-9.684301, -41.864103) knots 0 0 0 0 1 1 1 1
  spline S1204 degree 3 poles (-9.684301, -41.864103) (-9.540547, -41.159664) (-9.3411, -40.4714) (-9.085957, -39.799004) knots 0 0 0 0 1 1 1 1
  spline S1205 degree 3 poles (-9.085957, -39.799004) (-8.831125, -39.126919) (-8.523708, -38.479415) (-8.16433, -37.856804) knots 0 0 0 0 1 1 1 1
  spline S1206 degree 3 poles (-8.16433, -37.856804) (-7.80464, -37.234192) (-7.397656, -36.644562) (-6.943065, -36.087914) knots 0 0 0 0 1 1 1 1
  spline S1207 degree 3 poles (-6.943065, -36.087914) (-6.488164, -35.531266) (-5.991879, -35.014757) (-5.453899, -34.538386) knots 0 0 0 0 1 1 1 1
  spline S1208 degree 3 poles (-5.453899, -34.538386) (-5.413762, -34.500737) (-5.367089, -34.473978) (-5.314194, -34.458109) knots 0 0 0 0 1 1 1 1
  spline S1209 degree 3 poles (-5.314194, -34.458109) (-5.261609, -34.442552) (-5.208091, -34.43944) (-5.153642, -34.44877) knots 0 0 0 0 1 1 1 1
  spline S1210 degree 3 poles (-7.531452, -40.460504) (-7.512783, -40.463929) (-7.494737, -40.468594) (-7.47669, -40.474506) knots 0 0 0 0 1 1 1 1
  spline S1211 degree 3 poles (-7.47669, -40.474506) (-7.454909, -40.482287) (-7.434062, -40.491931) (-7.414149, -40.503443) knots 0 0 0 0 1 1 1 1
  spline S1212 degree 3 poles (-7.414149, -40.503443) (-7.394235, -40.515267) (-7.375565, -40.528646) (-7.358453, -40.544204) knots 0 0 0 0 1 1 1 1
  spline S1213 degree 3 poles (-7.358453, -40.544204) (-7.341339, -40.55945) (-7.325782, -40.576563) (-7.31178, -40.594921) knots 0 0 0 0 1 1 1 1
  spline S1214 degree 3 poles (-7.31178, -40.594921) (-7.297779, -40.613279) (-7.285955, -40.632882) (-7.275687, -40.653729) knots 0 0 0 0 1 1 1 1
  spline S1215 degree 3 poles (-7.275687, -40.653729) (-7.265731, -40.674576) (-7.257952, -40.696356) (-7.252662, -40.719068) knots 0 0 0 0 1 1 1 1
  spline S1216 degree 3 poles (-7.252662, -40.719068) (-7.246129, -40.741162) (-7.242705, -40.763876) (-7.24146, -40.786901) knots 0 0 0 0 1 1 1 1
  spline S1217 degree 3 poles (-7.241771, -40.78721) (-7.239907, -40.809926) (-7.241142, -40.832951) (-7.244264, -40.855976) knots 0 0 0 0 1 1 1 1
  spline S1218 degree 3 poles (-7.244575, -40.855974) (-7.247379, -40.87869) (-7.252977, -40.901093) (-7.260444, -40.922871) knots 0 0 0 0 1 1 1 1
  spline S1219 degree 3 poles (-7.260444, -40.922871) (-7.414154, -41.345105) (-7.528967, -41.777604) (-7.604887, -42.220368) knots 0 0 0 0 1 1 1 1
  spline S1220 degree 3 poles (-7.604887, -42.220368) (-7.608003, -42.243084) (-7.61329, -42.265487) (-7.620756, -42.287265) knots 0 0 0 0 1 1 1 1
  spline S1221 degree 3 poles (-7.620756, -42.287265) (-7.628221, -42.309048) (-7.637559, -42.330206) (-7.64907, -42.350118) knots 0 0 0 0 1 1 1 1
  spline S1222 degree 3 poles (-7.64907, -42.350118) (-7.660895, -42.370034) (-7.674274, -42.388703) (-7.689519, -42.406125) knots 0 0 0 0 1 1 1 1
  spline S1223 degree 3 poles (-7.689519, -42.406125) (-7.704767, -42.42324) (-7.721569, -42.439109) (-7.739614, -42.453108) knots 0 0 0 0 1 1 1 1
  spline S1224 degree 3 poles (-7.739614, -42.453108) (-7.757973, -42.467113) (-7.777576, -42.479247) (-7.798111, -42.489202) knots 0 0 0 0 1 1 1 1
  spline S1225 degree 3 poles (-7.798111, -42.489202) (-7.818959, -42.499472) (-7.840428, -42.507562) (-7.86283, -42.513472) knots 0 0 0 0 1 1 1 1
  spline S1226 degree 3 poles (-7.86283, -42.513472) (-7.884923, -42.519383) (-7.907637, -42.52312) (-7.930661, -42.524673) knots 0 0 0 0 1 1 1 1
  spline S1227 degree 3 poles (-7.930661, -42.524673) (-7.953687, -42.526229) (-7.976401, -42.525312) (-7.999425, -42.522497) knots 0 0 0 0 1 1 1 1
  spline S1228 degree 3 poles (-7.999425, -42.522497) (-8.022762, -42.520324) (-8.045476, -42.515968) (-8.067568, -42.50912) knots 0 0 0 0 1 1 1 1
  spline S1229 degree 3 poles (-8.067568, -42.50912) (-8.089971, -42.502277) (-8.11144, -42.493252) (-8.131665, -42.48205) knots 0 0 0 0 1 1 1 1
  spline S1230 degree 3 poles (-8.131665, -42.48205) (-8.152201, -42.470849) (-8.171181, -42.457469) (-8.188917, -42.442223) knots 0 0 0 0 1 1 1 1
  spline S1231 degree 3 poles (-8.188917, -42.442223) (-8.206652, -42.426977) (-8.222521, -42.410175) (-8.236834, -42.391817) knots 0 0 0 0 1 1 1 1
  spline S1232 degree 3 poles (-8.236834, -42.391817) (-8.250835, -42.373148) (-8.26297, -42.353234) (-8.273238, -42.332387) knots 0 0 0 0 1 1 1 1
  spline S1233 degree 3 poles (-8.273238, -42.332387) (-8.283195, -42.311229) (-8.290974, -42.289448) (-8.296575, -42.266734) knots 0 0 0 0 1 1 1 1
  spline S1234 degree 3 poles (-8.296575, -42.266734) (-8.302174, -42.24402) (-8.305287, -42.220995) (-8.305909, -42.197659) knots 0 0 0 0 1 1 1 1
  spline S1235 degree 3 poles (-8.305909, -42.197659) (-8.306841, -42.174323) (-8.304977, -42.151297) (-8.300927, -42.127336) knots 0 0 0 0 1 1 1 1
  spline S1236 degree 3 poles (-8.300927, -42.127336) (-8.220654, -41.638211) (-8.09526, -41.159973) (-7.925061, -40.693558) knots 0 0 0 0 1 1 1 1
  spline S1237 degree 3 poles (-7.925057, -40.692934) (-7.911371, -40.653731) (-7.891457, -40.617638) (-7.865009, -40.584967) knots 0 0 0 0 1 1 1 1
  spline S1238 degree 3 poles (-7.864383, -40.585276) (-7.838561, -40.552607) (-7.807135, -40.525537) (-7.771042, -40.504379) knots 0 0 0 0 1 1 1 1
  spline S1239 degree 3 poles (-7.770727, -40.504999) (-7.734948, -40.48291) (-7.696366, -40.468286) (-7.655294, -40.460818) knots 0 0 0 0 1 1 1 1
  spline S1240 degree 3 poles (-7.655294, -40.460818) (-7.613911, -40.453355) (-7.572839, -40.453355) (-7.531452, -40.460504) knots 0 0 0 0 1 1 1 1
  spline S1241 degree 3 poles (-4.018877, -35.328703) (-3.986206, -35.334303) (-3.955091, -35.344571) (-3.925532, -35.359195) knots 0 0 0 0 1 1 1 1
  spline S1242 degree 3 poles (-3.925532, -35.359195) (-3.895661, -35.37382) (-3.868591, -35.392177) (-3.844321, -35.41458) knots 0 0 0 0 1 1 1 1
  spline S1243 degree 3 poles (-3.844321, -35.41458) (-3.819741, -35.436672) (-3.798894, -35.461875) (-3.781469, -35.49019) knots 0 0 0 0 1 1 1 1
  spline S1244 degree 3 poles (-3.781469, -35.49019) (-3.764045, -35.518504) (-3.750976, -35.548375) (-3.741953, -35.580423) knots 0 0 0 0 1 1 1 1
  spline S1245 degree 3 poles (-3.741953, -35.580423) (-3.73293, -35.612472) (-3.728885, -35.644831) (-3.729196, -35.678124) knots 0 0 0 0 1 1 1 1
  spline S1246 degree 3 poles (-3.729196, -35.678124) (-3.729506, -35.711106) (-3.734174, -35.743466) (-3.74382, -35.775515) knots 0 0 0 0 1 1 1 1
  spline S1247 degree 3 poles (-3.74382, -35.775515) (-3.753154, -35.807252) (-3.766845, -35.837122) (-3.784581, -35.864815) knots 0 0 0 0 1 1 1 1
  spline S1248 degree 3 poles (-3.784581, -35.864815) (-3.802627, -35.892818) (-3.823786, -35.91771) (-3.848678, -35.939491) knots 0 0 0 0 1 1 1 1
  spline S1249 degree 3 poles (-3.848678, -35.939491) (-4.440797, -36.455067) (-4.977842, -37.022916) (-5.459503, -37.642727) knots 0 0 0 0 1 1 1 1
  spline S1250 degree 3 poles (-5.459503, -37.642727) (-5.941475, -38.26285) (-6.359038, -38.923422) (-6.712505, -39.624755) knots 0 0 0 0 1 1 1 1
  spline S1251 degree 3 poles (-6.712505, -39.624755) (-6.723085, -39.645291) (-6.735219, -39.664271) (-6.749532, -39.682318) knots 0 0 0 0 1 1 1 1
  spline S1252 degree 3 poles (-6.749532, -39.682318) (-6.763845, -39.700053) (-6.779713, -39.716544) (-6.797138, -39.731168) knots 0 0 0 0 1 1 1 1
  spline S1253 degree 3 poles (-6.797138, -39.731168) (-6.814562, -39.746103) (-6.833232, -39.758861) (-6.853145, -39.770062) knots 0 0 0 0 1 1 1 1
  spline S1254 degree 3 poles (-6.853145, -39.770062) (-6.87337, -39.781263) (-6.894217, -39.790287) (-6.915686, -39.797443) knots 0 0 0 0 1 1 1 1
  spline S1255 degree 3 poles (-6.915686, -39.797443) (-6.937466, -39.804604) (-6.959869, -39.809578) (-6.982584, -39.812378) knots 0 0 0 0 1 1 1 1
  spline S1256 degree 3 poles (-6.982584, -39.812378) (-7.005297, -39.814863) (-7.028012, -39.815492) (-7.050726, -39.813932) knots 0 0 0 0 1 1 1 1
  spline S1257 degree 3 poles (-7.050726, -39.813932) (-7.073439, -39.812067) (-7.095842, -39.808331) (-7.117934, -39.802108) knots 0 0 0 0 1 1 1 1
  spline S1258 degree 3 poles (-7.117934, -39.802108) (-7.140026, -39.795887) (-7.161184, -39.787795) (-7.18172, -39.777527) knots 0 0 0 0 1 1 1 1
  spline S1259 degree 3 poles (-7.18172, -39.777527) (-7.201944, -39.76757) (-7.221236, -39.755435) (-7.239282, -39.741434) knots 0 0 0 0 1 1 1 1
  spline S1260 degree 3 poles (-7.239282, -39.741434) (-7.25764, -39.727432) (-7.274131, -39.711874) (-7.289066, -39.69445) knots 0 0 0 0 1 1 1 1
  spline S1261 degree 3 poles (-7.289066, -39.69445) (-7.304002, -39.677337) (-7.317381, -39.658668) (-7.328894, -39.639065) knots 0 0 0 0 1 1 1 1
  spline S1262 degree 3 poles (-7.328894, -39.639065) (-7.340096, -39.619152) (-7.349741, -39.598305) (-7.356898, -39.576835) knots 0 0 0 0 1 1 1 1
  spline S1263 degree 3 poles (-7.356898, -39.576835) (-7.364361, -39.555055) (-7.369654, -39.532963) (-7.372766, -39.510249) knots 0 0 0 0 1 1 1 1
  spline S1264 degree 3 poles (-7.372766, -39.510249) (-7.375881, -39.487535) (-7.376502, -39.464821) (-7.375251, -39.441796) knots 0 0 0 0 1 1 1 1
  spline S1265 degree 3 poles (-7.375251, -39.441796) (-7.374009, -39.419082) (-7.370273, -39.396679) (-7.364672, -39.374587) knots 0 0 0 0 1 1 1 1
  spline S1266 degree 3 poles (-7.364672, -39.374587) (-7.358761, -39.352185) (-7.350982, -39.331026) (-7.341025, -39.310179) knots 0 0 0 0 1 1 1 1
  spline S1267 degree 3 poles (-7.341025, -39.310179) (-6.967333, -38.568086) (-6.52581, -37.868931) (-6.016147, -37.212715) knots 0 0 0 0 1 1 1 1
  spline S1268 degree 3 poles (-6.016147, -37.212715) (-5.506483, -36.556499) (-4.938322, -35.955668) (-4.311977, -35.409911) knots 0 0 0 0 1 1 1 1
  spline S1269 degree 3 poles (-4.311977, -35.409911) (-4.271838, -35.374751) (-4.226099, -35.35017) (-4.174759, -35.335857) knots 0 0 0 0 1 1 1 1
  spline S1270 degree 3 poles (-4.174759, -35.335857) (-4.12342, -35.321544) (-4.071458, -35.319055) (-4.018877, -35.328703) knots 0 0 0 0 1 1 1 1
  spline S1271 degree 3 poles (-6.790604, -34.1566) (-6.72744, -34.167801) (-6.671433, -34.19456) (-6.622583, -34.236254) knots 0 0 0 0 1 1 1 1
  spline S1272 degree 3 poles (-6.622583, -34.236254) (-6.574043, -34.278259) (-6.539506, -34.329599) (-6.51897, -34.390585) knots 0 0 0 0 1 1 1 1
  spline S1273 degree 3 poles (-6.51897, -34.390585) (-6.498433, -34.45157) (-6.4947, -34.513489) (-6.50808, -34.576341) knots 0 0 0 0 1 1 1 1
  spline S1274 degree 3 poles (-6.50808, -34.576341) (-6.521459, -34.639194) (-6.550085, -34.694578) (-6.593646, -34.741873) knots 0 0 0 0 1 1 1 1
  spline S1275 degree 3 poles (-6.593646, -34.741873) (-7.406681, -35.666301) (-8.152197, -36.64269) (-8.830194, -37.670731) knots 0 0 0 0 1 1 1 1
  spline S1276 degree 3 poles (-8.830194, -37.670731) (-8.849485, -37.701535) (-8.873132, -37.728605) (-8.900825, -37.75163) knots 0 0 0 0 1 1 1 1
  spline S1277 degree 3 poles (-8.900825, -37.75163) (-8.928828, -37.774966) (-8.959632, -37.793013) (-8.993548, -37.806392) knots 0 0 0 0 1 1 1 1
  spline S1278 degree 3 poles (-8.993548, -37.806392) (-9.027152, -37.819772) (-9.062001, -37.82724) (-9.098405, -37.829418) knots 0 0 0 0 1 1 1 1
  spline S1279 degree 3 poles (-9.098405, -37.829418) (-9.134499, -37.831282) (-9.16997, -37.827864) (-9.20513, -37.818527) knots 0 0 0 0 1 1 1 1
  spline S1280 degree 3 poles (-9.20513, -37.818527) (-9.24029, -37.810126) (-9.273583, -37.796436) (-9.304387, -37.777767) knots 0 0 0 0 1 1 1 1
  spline S1281 degree 3 poles (-9.304387, -37.777767) (-9.335502, -37.759098) (-9.363195, -37.736072) (-9.387153, -37.709002) knots 0 0 0 0 1 1 1 1
  spline S1282 degree 3 poles (-9.387153, -37.709002) (-9.411111, -37.681932) (-9.430403, -37.651751) (-9.445027, -37.618458) knots 0 0 0 0 1 1 1 1
  spline S1283 degree 3 poles (-9.445027, -37.618458) (-9.459651, -37.585165) (-9.468985, -37.550627) (-9.47303, -37.514533) knots 0 0 0 0 1 1 1 1
  spline S1284 degree 2 poles (-9.47303, -37.514533) (-9.534327, -36.957886) (-9.611803, -36.432042) knots 0 0 0 1 1 1
  line L25 (-9.611803, -36.432042) -> (-9.790092, -35.029998)
  spline S1285 degree 3 poles (-9.790092, -35.029998) (-9.792896, -35.007284) (-9.793517, -34.984259) (-9.791957, -34.960923) knots 0 0 0 0 1 1 1 1
  spline S1286 degree 3 poles (-9.791957, -34.960923) (-9.790403, -34.937898) (-9.786667, -34.915184) (-9.780755, -34.893092) knots 0 0 0 0 1 1 1 1
  spline S1287 degree 3 poles (-9.780755, -34.893092) (-9.774535, -34.870689) (-9.766442, -34.84922) (-9.756175, -34.828373) knots 0 0 0 0 1 1 1 1
  spline S1288 degree 3 poles (-9.756175, -34.828373) (-9.745907, -34.807526) (-9.733461, -34.788235) (-9.719459, -34.769877) knots 0 0 0 0 1 1 1 1
  spline S1289 degree 3 poles (-9.719459, -34.769877) (-9.705457, -34.751519) (-9.689588, -34.734717) (-9.672164, -34.71947) knots 0 0 0 0 1 1 1 1
  spline S1290 degree 3 poles (-9.672164, -34.71947) (-9.65474, -34.704224) (-9.63607, -34.691156) (-9.615846, -34.679643) knots 0 0 0 0 1 1 1 1
  spline S1291 degree 3 poles (-9.615846, -34.679643) (-9.595932, -34.668131) (-9.574774, -34.658485) (-9.552993, -34.651329) knots 0 0 0 0 1 1 1 1
  spline S1292 degree 3 poles (-9.552993, -34.651329) (-9.531213, -34.643866) (-9.50881, -34.638571) (-9.485785, -34.635771) knots 0 0 0 0 1 1 1 1
  spline S1293 degree 3 poles (-9.485785, -34.635771) (-9.46276, -34.632657) (-9.439735, -34.632035) (-9.41671, -34.633595) knots 0 0 0 0 1 1 1 1
  spline S1294 degree 3 poles (-9.41671, -34.633595) (-9.393684, -34.635149) (-9.37097, -34.638885) (-9.348879, -34.645108) knots 0 0 0 0 1 1 1 1
  spline S1295 degree 3 poles (-9.348879, -34.645108) (-9.326476, -34.651017) (-9.305007, -34.659421) (-9.284471, -34.669689) knots 0 0 0 0 1 1 1 1
  spline S1296 degree 3 poles (-9.284471, -34.669689) (-9.263625, -34.679957) (-9.244021, -34.692092) (-9.225974, -34.706093) knots 0 0 0 0 1 1 1 1
  spline S1297 degree 3 poles (-9.225974, -34.706093) (-9.207617, -34.720406) (-9.190814, -34.736275) (-9.175568, -34.753699) knots 0 0 0 0 1 1 1 1
  spline S1298 degree 3 poles (-9.175568, -34.753699) (-9.160633, -34.771124) (-9.147253, -34.789793) (-9.135741, -34.809706) knots 0 0 0 0 1 1 1 1
  spline S1299 degree 3 poles (-9.135741, -34.809706) (-9.124228, -34.829931) (-9.114894, -34.850778) (-9.107426, -34.87287) knots 0 0 0 0 1 1 1 1
  spline S1300 degree 3 poles (-9.107426, -34.87287) (-9.099962, -34.89465) (-9.09498, -34.917364) (-9.091869, -34.940078) knots 0 0 0 0 1 1 1 1
  line L26 (-9.091869, -34.940078) -> (-8.912646, -36.335899)
  spline S1301 degree 3 poles (-8.912646, -36.335899) (-8.903622, -36.394084) (-8.894911, -36.452891) (-8.886821, -36.511387) knots 0 0 0 0 1 1 1 1
  spline S1302 degree 3 poles (-8.886821, -36.511387) (-8.340441, -35.726978) (-7.749566, -34.977728) (-7.114198, -34.264877) knots 0 0 0 0 1 1 1 1
  spline S1303 degree 3 poles (-7.114198, -34.264877) (-7.072814, -34.219454) (-7.023652, -34.187717) (-6.96609, -34.168426) knots 0 0 0 0 1 1 1 1
  spline S1304 degree 3 poles (-6.96609, -34.168426) (-6.908527, -34.149446) (-6.850031, -34.145401) (-6.790604, -34.1566) knots 0 0 0 0 1 1 1 1
  line L27 (-21.591027, -44.735505) -> (-17.573455, -44.735505)
  spline S1305 degree 3 poles (-17.573455, -44.735505) (-16.906038, -44.735505) (-16.251377, -44.194104) (-16.251377, -43.520463) knots 0 0 0 0 1 1 1 1
  line L28 (-16.251377, -43.520463) -> (-16.251377, -43.293635)